Autodesk Fusion 360 part; units mm, degrees
note: some values were not read from the file. Set by a fixed rule: which sketch regions a step uses.
(part 8 of 8)
  spline S20 degree 5 poles (-1.278, 13.0935) (-1.2788, 13.1018) (-1.2807, 13.1185) (-1.2843, 13.1435) (-1.2905, 13.1765) (-1.3001, 13.2175) (-1.3112, 13.2582) (-1.3231, 13.2988) (-1.3355, 13.3394) (-1.3483, 13.3799) (-1.3613, 13.4204) (-1.3749, 13.4608) (-1.389, 13.5011) (-1.4038, 13.5413) (-1.4192, 13.5813) (-1.4354, 13.6213) (-1.452, 13.6611) (-1.4691, 13.7008) (-1.4866, 13.7404) (-1.5045, 13.7799) (-1.5227, 13.8194) (-1.5414, 13.8588) (-1.5605, 13.898) (-1.58, 13.9372) (-1.5999, 13.9763) (-1.6202, 14.0152) (-1.6409, 14.0541) (-1.662, 14.0929) (-1.6834, 14.1316) (-1.7052, 14.1701) (-1.7274, 14.2086) (-1.7498, 14.247) (-1.7726, 14.2853) (-1.7958, 14.3235) (-1.8193, 14.3616) (-1.8431, 14.3996) (-1.8673, 14.4374) (-1.8918, 14.4752) (-1.9166, 14.5129) (-1.9417, 14.5505) (-1.9671, 14.588) (-1.9928, 14.6254) (-2.0188, 14.6626) (-2.0451, 14.6998) (-2.0717, 14.7369) (-2.0987, 14.7738) (-2.1259, 14.8107) (-2.1534, 14.8474) (-2.1811, 14.8841) (-2.2092, 14.9206) (-2.2375, 14.957) (-2.2662, 14.9934) (-2.2951, 15.0296) (-2.3242, 15.0657) (-2.3537, 15.1017) (-2.3834, 15.1375) (-2.4134, 15.1733) (-2.4436, 15.2089) (-2.4741, 15.2445) (-2.5049, 15.2799) (-2.5359, 15.3152) (-2.5672, 15.3504) (-2.5987, 15.3855) (-2.6305, 15.4205) (-2.6626, 15.4553) (-2.6949, 15.4901) (-2.7274, 15.5247) (-2.7602, 15.5592) (-2.7932, 15.5936) (-2.8265, 15.6278) (-2.86, 15.662) (-2.887, 15.6892) (-2.9074, 15.7095) (-2.921, 15.7231) (-2.9278, 15.7298) knots 0 0 0 0 0 0 0.01428571 0.02857143 0.04285714 0.05714286 0.07142857 0.08571429 0.1 0.11428571 0.12857143 0.14285714 0.15714286 0.17142857 0.18571429 0.2 0.21428571 0.22857143 0.24285714 0.25714286 0.27142857 0.28571429 0.3 0.31428571 0.32857143 0.34285714 0.35714286 0.37142857 0.38571429 0.4 0.41428571 0.42857143 0.44285714 0.45714286 0.47142857 0.48571429 0.5 0.51428571 0.52857143 0.54285714 0.55714286 0.57142857 0.58571429 0.6 0.61428571 0.62857143 0.64285714 0.65714286 0.67142857 0.68571429 0.7 0.71428571 0.72857143 0.74285714 0.75714286 0.77142857 0.78571429 0.8 0.81428571 0.82857143 0.84285714 0.85714286 0.87142857 0.88571429 0.9 0.91428571 0.92857143 0.94285714 0.95714286 0.97142857 0.98571429 1 1 1 1 1 1
  arc A43 (-2.9278, 15.7298) -> (-4.187, 15.4424) centre (0, 0) ccw
  spline S21 degree 5 poles (-4.187, 15.4424) (-4.1903, 15.4334) (-4.1967, 15.4153) (-4.2062, 15.3881) (-4.2187, 15.3518) (-4.2341, 15.3065) (-4.2492, 15.2612) (-4.264, 15.2159) (-4.2786, 15.1706) (-4.2929, 15.1253) (-4.3069, 15.08) (-4.3207, 15.0347) (-4.3342, 14.9894) (-4.3473, 14.9441) (-4.3603, 14.8988) (-4.3729, 14.8536) (-4.3852, 14.8083) (-4.3973, 14.763) (-4.4091, 14.7178) (-4.4206, 14.6726) (-4.4318, 14.6273) (-4.4427, 14.5821) (-4.4533, 14.537) (-4.4636, 14.4918) (-4.4737, 14.4467) (-4.4834, 14.4015) (-4.4928, 14.3564) (-4.502, 14.3114) (-4.5108, 14.2663) (-4.5193, 14.2213) (-4.5275, 14.1764) (-4.5354, 14.1314) (-4.543, 14.0865) (-4.5503, 14.0416) (-4.5572, 13.9968) (-4.5639, 13.952) (-4.5702, 13.9072) (-4.5761, 13.8625) (-4.5818, 13.8179) (-4.5871, 13.7733) (-4.5921, 13.7287) (-4.5968, 13.6842) (-4.6011, 13.6397) (-4.605, 13.5953) (-4.6086, 13.551) (-4.6118, 13.5067) (-4.6147, 13.4625) (-4.6172, 13.4184) (-4.6194, 13.3743) (-4.6212, 13.3303) (-4.6226, 13.2864) (-4.6236, 13.2425) (-4.6242, 13.1988) (-4.6243, 13.1551) (-4.6241, 13.1115) (-4.6234, 13.0681) (-4.6223, 13.0247) (-4.6209, 12.9814) (-4.6191, 12.9382) (-4.6168, 12.8951) (-4.614, 12.8521) (-4.6106, 12.8094) (-4.6065, 12.7667) (-4.6017, 12.7243) (-4.5964, 12.682) (-4.5906, 12.6399) (-4.5845, 12.5979) (-4.5781, 12.5559) (-4.5712, 12.5141) (-4.5635, 12.4726) (-4.5544, 12.4315) (-4.5457, 12.3991) (-4.5381, 12.3751) (-4.5325, 12.3592) (-4.5296, 12.3513) knots -1 -1 -1 -1 -1 -1 -0.98571429 -0.97142857 -0.95714286 -0.94285714 -0.92857143 -0.91428571 -0.9 -0.88571429 -0.87142857 -0.85714286 -0.84285714 -0.82857143 -0.81428571 -0.8 -0.78571429 -0.77142857 -0.75714286 -0.74285714 -0.72857143 -0.71428571 -0.7 -0.68571429 -0.67142857 -0.65714286 -0.64285714 -0.62857143 -0.61428571 -0.6 -0.58571429 -0.57142857 -0.55714286 -0.54285714 -0.52857143 -0.51428571 -0.5 -0.48571429 -0.47142857 -0.45714286 -0.44285714 -0.42857143 -0.41428571 -0.4 -0.38571429 -0.37142857 -0.35714286 -0.34285714 -0.32857143 -0.31428571 -0.3 -0.28571429 -0.27142857 -0.25714286 -0.24285714 -0.22857143 -0.21428571 -0.2 -0.18571429 -0.17142857 -0.15714286 -0.14285714 -0.12857143 -0.11428571 -0.1 -0.08571429 -0.07142857 -0.05714286 -0.04285714 -0.02857143 -0.01428571 0 0 0 0 0 0
  line L23 (-4.5296, 12.3513) -> (-4.3545, 11.8727)
  arc A44 (-4.9424, 10.4382) -> (-4.3545, 11.8727) centre (-5.4345, 11.4776) ccw
  arc A45 (-4.9424, 10.4382) -> (-5.0794, 10.3723) centre (0, 0) ccw
  arc A46 (-6.5675, 10.807) -> (-5.0794, 10.3723) centre (-5.5852, 11.4051) ccw
  line L24 (-6.5675, 10.807) -> (-6.8325, 11.2423)
  spline S22 degree 5 poles (-6.8325, 11.2423) (-6.8368, 11.2495) (-6.8458, 11.2637) (-6.8598, 11.2846) (-6.8797, 11.3117) (-6.9062, 11.3444) (-6.9339, 11.3763) (-6.9622, 11.4078) (-6.991, 11.4389) (-7.0201, 11.4699) (-7.0494, 11.5007) (-7.0791, 11.5313) (-7.1093, 11.5614) (-7.1401, 11.5912) (-7.1714, 11.6206) (-7.2032, 11.6495) (-7.2355, 11.6782) (-7.2682, 11.7065) (-7.3011, 11.7347) (-7.3344, 11.7625) (-7.368, 11.7902) (-7.4018, 11.8175) (-7.4361, 11.8446) (-7.4706, 11.8715) (-7.5055, 11.898) (-7.5407, 11.9243) (-7.5763, 11.9503) (-7.6121, 11.9761) (-7.6482, 12.0017) (-7.6846, 12.027) (-7.7212, 12.0521) (-7.7581, 12.0769) (-7.7953, 12.1015) (-7.8327, 12.1258) (-7.8704, 12.15) (-7.9083, 12.1739) (-7.9465, 12.1975) (-7.985, 12.2209) (-8.0237, 12.2441) (-8.0626, 12.2671) (-8.1018, 12.2898) (-8.1411, 12.3124) (-8.1808, 12.3347) (-8.2206, 12.3567) (-8.2607, 12.3786) (-8.301, 12.4002) (-8.3415, 12.4216) (-8.3822, 12.4428) (-8.4231, 12.4637) (-8.4642, 12.4845) (-8.5056, 12.505) (-8.5471, 12.5253) (-8.5889, 12.5454) (-8.6308, 12.5653) (-8.6729, 12.5849) (-8.7153, 12.6043) (-8.7578, 12.6236) (-8.8005, 12.6426) (-8.8434, 12.6613) (-8.8865, 12.6799) (-8.9298, 12.6983) (-8.9733, 12.7164) (-9.0169, 12.7343) (-9.0607, 12.752) (-9.1047, 12.7695) (-9.1489, 12.7868) (-9.1932, 12.8039) (-9.2377, 12.8207) (-9.2824, 12.8374) (-9.3272, 12.8538) (-9.3722, 12.87) (-9.4084, 12.8828) (-9.4356, 12.8923) (-9.4537, 12.8986) (-9.4628, 12.9018) knots 0 0 0 0 0 0 0.01428571 0.02857143 0.04285714 0.05714286 0.07142857 0.08571429 0.1 0.11428571 0.12857143 0.14285714 0.15714286 0.17142857 0.18571429 0.2 0.21428571 0.22857143 0.24285714 0.25714286 0.27142857 0.28571429 0.3 0.31428571 0.32857143 0.34285714 0.35714286 0.37142857 0.38571429 0.4 0.41428571 0.42857143 0.44285714 0.45714286 0.47142857 0.48571429 0.5 0.51428571 0.52857143 0.54285714 0.55714286 0.57142857 0.58571429 0.6 0.61428571 0.62857143 0.64285714 0.65714286 0.67142857 0.68571429 0.7 0.71428571 0.72857143 0.74285714 0.75714286 0.77142857 0.78571429 0.8 0.81428571 0.82857143 0.84285714 0.85714286 0.87142857 0.88571429 0.9 0.91428571 0.92857143 0.94285714 0.95714286 0.97142857 0.98571429 1 1 1 1 1 1
  arc A47 (-9.4628, 12.9018) -> (-10.4726, 12.0965) centre (0, 0) ccw
  spline S23 degree 5 poles (-10.4726, 12.0965) (-10.4716, 12.0869) (-10.4695, 12.0678) (-10.4663, 12.0392) (-10.4618, 12.0011) (-10.456, 11.9536) (-10.45, 11.9062) (-10.4437, 11.859) (-10.4372, 11.8118) (-10.4304, 11.7648) (-10.4234, 11.7179) (-10.4161, 11.6711) (-10.4086, 11.6245) (-10.4008, 11.5779) (-10.3928, 11.5315) (-10.3846, 11.4853) (-10.376, 11.4391) (-10.3673, 11.3931) (-10.3583, 11.3472) (-10.349, 11.3015) (-10.3395, 11.2559) (-10.3297, 11.2104) (-10.3196, 11.1651) (-10.3094, 11.12) (-10.2988, 11.0749) (-10.288, 11.0301) (-10.2769, 10.9854) (-10.2656, 10.9408) (-10.254, 10.8964) (-10.2422, 10.8521) (-10.23, 10.808) (-10.2177, 10.7641) (-10.205, 10.7204) (-10.1921, 10.6768) (-10.1789, 10.6334) (-10.1654, 10.5901) (-10.1517, 10.5471) (-10.1377, 10.5042) (-10.1234, 10.4615) (-10.1089, 10.419) (-10.094, 10.3767) (-10.0789, 10.3346) (-10.0635, 10.2926) (-10.0478, 10.2509) (-10.0318, 10.2094) (-10.0155, 10.1681) (-9.9989, 10.1271) (-9.982, 10.0862) (-9.9648, 10.0455) (-9.9474, 10.0051) (-9.9296, 9.9649) (-9.9115, 9.925) (-9.893, 9.8853) (-9.8742, 9.8459) (-9.855, 9.8068) (-9.8356, 9.7679) (-9.8158, 9.7293) (-9.7957, 9.6909) (-9.7753, 9.6528) (-9.7546, 9.6149) (-9.7334, 9.5774) (-9.7118, 9.5404) (-9.6896, 9.5038) (-9.6669, 9.4676) (-9.6437, 9.4318) (-9.6202, 9.3964) (-9.5965, 9.3611) (-9.5725, 9.3261) (-9.5482, 9.2915) (-9.5232, 9.2574) (-9.4972, 9.2243) (-9.4753, 9.1989) (-9.458, 9.1806) (-9.4461, 9.1687) (-9.4401, 9.1628) knots -1 -1 -1 -1 -1 -1 -0.98571429 -0.97142857 -0.95714286 -0.94285714 -0.92857143 -0.91428571 -0.9 -0.88571429 -0.87142857 -0.85714286 -0.84285714 -0.82857143 -0.81428571 -0.8 -0.78571429 -0.77142857 -0.75714286 -0.74285714 -0.72857143 -0.71428571 -0.7 -0.68571429 -0.67142857 -0.65714286 -0.64285714 -0.62857143 -0.61428571 -0.6 -0.58571429 -0.57142857 -0.55714286 -0.54285714 -0.52857143 -0.51428571 -0.5 -0.48571429 -0.47142857 -0.45714286 -0.44285714 -0.42857143 -0.41428571 -0.4 -0.38571429 -0.37142857 -0.35714286 -0.34285714 -0.32857143 -0.31428571 -0.3 -0.28571429 -0.27142857 -0.25714286 -0.24285714 -0.22857143 -0.21428571 -0.2 -0.18571429 -0.17142857 -0.15714286 -0.14285714 -0.12857143 -0.11428571 -0.1 -0.08571429 -0.07142857 -0.05714286 -0.04285714 -0.02857143 -0.01428571 0 0 0 0 0 0
  line L25 (-9.4401, 9.1628) -> (-9.0747, 8.8076)
  arc A48 (-8.9819, 7.2601) -> (-9.0747, 8.8076) centre (-9.8763, 7.983) ccw
  arc A49 (-8.9819, 7.2601) -> (-9.0767, 7.1412) centre (0, 0) ccw
  arc A50 (-10.6061, 6.8873) -> (-9.0767, 7.1412) centre (-9.9805, 7.8523) ccw
  line L26 (-10.6061, 6.8873) -> (-11.0337, 7.1645)
  spline S24 degree 5 poles (-11.0337, 7.1645) (-11.0408, 7.1691) (-11.055, 7.178) (-11.0767, 7.1907) (-11.1064, 7.2065) (-11.1444, 7.2245) (-11.1832, 7.2412) (-11.2224, 7.2572) (-11.2619, 7.2728) (-11.3015, 7.2882) (-11.3413, 7.3032) (-11.3813, 7.3178) (-11.4216, 7.3319) (-11.4622, 7.3453) (-11.5032, 7.3582) (-11.5444, 7.3705) (-11.586, 7.3823) (-11.6277, 7.3937) (-11.6696, 7.4047) (-11.7116, 7.4154) (-11.7539, 7.4257) (-11.7963, 7.4357) (-11.8389, 7.4453) (-11.8816, 7.4544) (-11.9246, 7.4632) (-11.9677, 7.4716) (-12.011, 7.4797) (-12.0545, 7.4874) (-12.0981, 7.4947) (-12.1419, 7.5017) (-12.1857, 7.5084) (-12.2298, 7.5148) (-12.2739, 7.5208) (-12.3182, 7.5265) (-12.3626, 7.5319) (-12.4072, 7.537) (-12.4519, 7.5417) (-12.4967, 7.5461) (-12.5416, 7.5502) (-12.5866, 7.554) (-12.6318, 7.5575) (-12.677, 7.5607) (-12.7224, 7.5636) (-12.7679, 7.5662) (-12.8135, 7.5685) (-12.8591, 7.5705) (-12.9049, 7.5722) (-12.9508, 7.5737) (-12.9968, 7.5748) (-13.0428, 7.5756) (-13.089, 7.5762) (-13.1352, 7.5764) (-13.1815, 7.5764) (-13.2279, 7.5761) (-13.2744, 7.5756) (-13.321, 7.5747) (-13.3677, 7.5736) (-13.4144, 7.5721) (-13.4612, 7.5704) (-13.5081, 7.5685) (-13.555, 7.5662) (-13.6021, 7.5637) (-13.6492, 7.5609) (-13.6963, 7.5579) (-13.7435, 7.5546) (-13.7908, 7.551) (-13.8382, 7.5471) (-13.8856, 7.543) (-13.9331, 7.5386) (-13.9806, 7.5339) (-14.0282, 7.529) (-14.0663, 7.5249) (-14.0949, 7.5217) (-14.114, 7.5194) (-14.1236, 7.5183) knots 0 0 0 0 0 0 0.01428571 0.02857143 0.04285714 0.05714286 0.07142857 0.08571429 0.1 0.11428571 0.12857143 0.14285714 0.15714286 0.17142857 0.18571429 0.2 0.21428571 0.22857143 0.24285714 0.25714286 0.27142857 0.28571429 0.3 0.31428571 0.32857143 0.34285714 0.35714286 0.37142857 0.38571429 0.4 0.41428571 0.42857143 0.44285714 0.45714286 0.47142857 0.48571429 0.5 0.51428571 0.52857143 0.54285714 0.55714286 0.57142857 0.58571429 0.6 0.61428571 0.62857143 0.64285714 0.65714286 0.67142857 0.68571429 0.7 0.71428571 0.72857143 0.74285714 0.75714286 0.77142857 0.78571429 0.8 0.81428571 0.82857143 0.84285714 0.85714286 0.87142857 0.88571429 0.9 0.91428571 0.92857143 0.94285714 0.95714286 0.97142857 0.98571429 1 1 1 1 1 1
  arc A51 (-14.1236, 7.5183) -> (-14.684, 6.3546) centre (0, 0) ccw
  spline S25 degree 5 poles (-14.684, 6.3546) (-14.6789, 6.3465) (-14.6687, 6.3302) (-14.6534, 6.3058) (-14.6329, 6.2734) (-14.607, 6.2331) (-14.581, 6.1931) (-14.5549, 6.1532) (-14.5285, 6.1136) (-14.502, 6.0741) (-14.4754, 6.0349) (-14.4485, 5.9959) (-14.4215, 5.9572) (-14.3943, 5.9186) (-14.367, 5.8803) (-14.3394, 5.8422) (-14.3117, 5.8043) (-14.2839, 5.7666) (-14.2558, 5.7292) (-14.2276, 5.692) (-14.1993, 5.6551) (-14.1707, 5.6184) (-14.142, 5.5819) (-14.1132, 5.5457) (-14.0841, 5.5097) (-14.0549, 5.474) (-14.0256, 5.4385) (-13.996, 5.4032) (-13.9663, 5.3683) (-13.9364, 5.3335) (-13.9064, 5.2991) (-13.8762, 5.2649) (-13.8458, 5.2309) (-13.8152, 5.1973) (-13.7845, 5.1639) (-13.7536, 5.1308) (-13.7226, 5.0979) (-13.6914, 5.0654) (-13.66, 5.0331) (-13.6284, 5.0011) (-13.5967, 4.9694) (-13.5648, 4.9381) (-13.5327, 4.907) (-13.5004, 4.8762) (-13.468, 4.8458) (-13.4354, 4.8156) (-13.4026, 4.7858) (-13.3697, 4.7563) (-13.3366, 4.7271) (-13.3033, 4.6983) (-13.2699, 4.6698) (-13.2362, 4.6417) (-13.2024, 4.6139) (-13.1683, 4.5866) (-13.1341, 4.5597) (-13.0997, 4.5331) (-13.0651, 4.5069) (-13.0304, 4.481) (-12.9954, 4.4555) (-12.9603, 4.4304) (-12.925, 4.4058) (-12.8894, 4.3818) (-12.8535, 4.3584) (-12.8174, 4.3357) (-12.781, 4.3135) (-12.7445, 4.2918) (-12.7078, 4.2703) (-12.671, 4.2492) (-12.634, 4.2285) (-12.5968, 4.2087) (-12.559, 4.1902) (-12.5282, 4.1768) (-12.5047, 4.1677) (-12.4888, 4.1622) (-12.4808, 4.1595) knots -1 -1 -1 -1 -1 -1 -0.98571429 -0.97142857 -0.95714286 -0.94285714 -0.92857143 -0.91428571 -0.9 -0.88571429 -0.87142857 -0.85714286 -0.84285714 -0.82857143 -0.81428571 -0.8 -0.78571429 -0.77142857 -0.75714286 -0.74285714 -0.72857143 -0.71428571 -0.7 -0.68571429 -0.67142857 -0.65714286 -0.64285714 -0.62857143 -0.61428571 -0.6 -0.58571429 -0.57142857 -0.55714286 -0.54285714 -0.52857143 -0.51428571 -0.5 -0.48571429 -0.47142857 -0.45714286 -0.44285714 -0.42857143 -0.41428571 -0.4 -0.38571429 -0.37142857 -0.35714286 -0.34285714 -0.32857143 -0.31428571 -0.3 -0.28571429 -0.27142857 -0.25714286 -0.24285714 -0.22857143 -0.21428571 -0.2 -0.18571429 -0.17142857 -0.15714286 -0.14285714 -0.12857143 -0.11428571 -0.1 -0.08571429 -0.07142857 -0.05714286 -0.04285714 -0.02857143 -0.01428571 0 0 0 0 0 0
  line L27 (-12.4808, 4.1595) -> (-11.9975, 3.998)
  arc A52 (-11.2425, 2.644) -> (-11.9975, 3.998) centre (-12.3619, 2.9073) ccw
  circle A53 centre (0, 0) radius 1.5
  circle A54 centre (0, 0) radius 11.5492
  line L28 (-5.4205, -10.2669) -> (-5.4065, -10.2056)
  constraint concentric A1 A54
  constraint coincident A8.start A54
  constraint coincident A12.start L6.start
  constraint coincident A54 L28.end
  constraint parallel L6 L28
extrude "Extrude5" cut sketch "Sketch7" against normal blind 5 contours A50 L26 S24 A51 S25 L27 A52 A54 | A2 L0 S0 A3 S1 L1 A4 A54 | A46 L24 S22 A47 S23 L25 A48 A54 | A6 L2 S2 A7 S3 L3 A8 A54 | A42 L22 S20 A43 S21 L23 A44 A54 | A10 L4 S4 A11 S5 L5 A12 A54 L28 bodies 4 in component "Spur Gear (14 teeth) (1)"
sketch "Sketch1 (4)" plane through (0, 0, 0) normal (0, 0, 1) x (-1, 0, 0) in component "Gripper (1)"
  circle A0 centre (-11, -59.5) radius 1.5
  circle A1 centre (-11, -35.5) radius 1.5
  arc A2 (-8, -35.5) -> (-14, -35.5) centre (-11, -35.5) ccw
  line L0 (-14, -35.5) -> (-14, -59.5)
  arc A3 (-14, -59.5) -> (-8, -59.5) centre (-11, -59.5) ccw
  line L1 (-8, -59.5) -> (-8, -35.5)
  circle A4 centre (-11, -59.5) radius 1.5
  circle A5 centre (-19, -77.8303) radius 1.5
  line L2 (-13.7495, -58.3) -> (-21.7495, -76.6303)
  arc A6 (-21.7495, -76.6303) -> (-16.2505, -79.0303) centre (-19, -77.8303) ccw
  line L3 (-16.2505, -79.0303) -> (-8.2505, -60.7)
  arc A7 (-8.2505, -60.7) -> (-13.7495, -58.3) centre (-11, -59.5) ccw
  line L4 (-11, -59.5) -> (-19, -77.8303) construction
  line L5 (-17.5, -77.8303) -> (-25, -77.8303)
  line L6 (-25, -77.8303) -> (-25, -102.8303)
  line L7 (-25, -102.8303) -> (-17.5, -102.8303)
  line L8 (-17.5, -102.8303) -> (-17.5, -77.8303)
  dimension "d32_1" = 6
  dimension "d33_1" = 25
  dimension "d34_1" = 6
  constraint tangent L2 A6
  constraint tangent A6 L3
  constraint parallel L2 L3
  constraint tangent L3 A7
  constraint tangent L2 A7
  constraint coincident A5.centre A6.centre
  constraint coincident A0.centre A3.centre
  constraint horizontal L5
  constraint vertical L6
  constraint horizontal L7
  constraint vertical L8
  constraint coincident A5 L5.start
  measures "d32_1" diameter of A6
  measures "d33_1" distance of L5.end L6.end
  measures "d34_1" distance of A5.centre L6
extrude "Extrude1''''" add sketch "Sketch1 (4)" along normal blind 5 separate body contours L0 A3 L2 A7 | L0 A3 A5 L2 A6 L3 L5 L8 | A5 A6 L5 L8 | A6 L5 L6 L7 L8 makes body 5 in component "Gripper (1)"
fillet "Fillet1''" radius 6 2 edges at (17.5, 80.4284, 2.5) (17.5, 102.8303, 2.5) on bodies 5 in component "Gripper (1)"
fillet "Fillet2" radius 6 1 edges at (22, 77.8303, 2.5) on bodies 5 in component "Gripper (1)"
component "MotorBase" placed x (1, 0, 0) y (0, 1, 0) z (0, 0, 1) at (0, 0, 0)
component "Link" placed x (0.475457, 0.879739, 0) y (-0.879739, 0.475457, 0) z (0, 0, 1) at (24.6989, 48.1344, -10)
component "Link" placed x (0.475457, 0.879739, 0) y (-0.879739, 0.475457, 0) z (0, 0, 1) at (32.6989, 66.4647, -10)
component "Link" placed x (0.475457, 0.879739, 0) y (-0.879739, 0.475457, 0) z (0, 0, 1) at (32.6989, 66.4647, 0)
component "Link" placed x (0.798992, -0.601341, 0) y (0.601341, 0.798992, 0) z (0, 0, 1) at (41.4501, 38.4004, -10)
component "Link" placed x (0.798992, -0.601341, 0) y (0.601341, 0.798992, 0) z (0, 0, 1) at (41.4501, 38.4004, 0)
component "Link" placed x (0.798992, -0.601341, 0) y (0.601341, 0.798992, 0) z (0, 0, 1) at (49.4501, 20.0701, -10)
component "Spur Gear (14 teeth)" placed x (0.797282, 0.603607, 0) y (-0.603607, 0.797282, 0) z (0, 0, 1) at (11, 35.5, 5)
component "Spur Gear (14 teeth) (1)" placed x (0.912771, -0.408472, 0) y (0.408472, 0.912771, 0) z (0, 0, 1) at (39, 35.5, 5)
component "Gripper (1)" placed x (1, 0, 0) y (0, 1, 0) z (0, 0, 1) at (-2.0885, 9.5142, -7.6495)
component "Gripper (1)" placed x (-1, 0, 0) y (0, 1, 0) z (0, 0, -1) at (54.1972, 9.5142, -2.6495)
equation "taperAngle1 = 0.0 deg"
equation "Radius = 1.15 mm"
equation "countU = 14"
equation "d104 = ( 360 / 28 ) * 1 deg"
